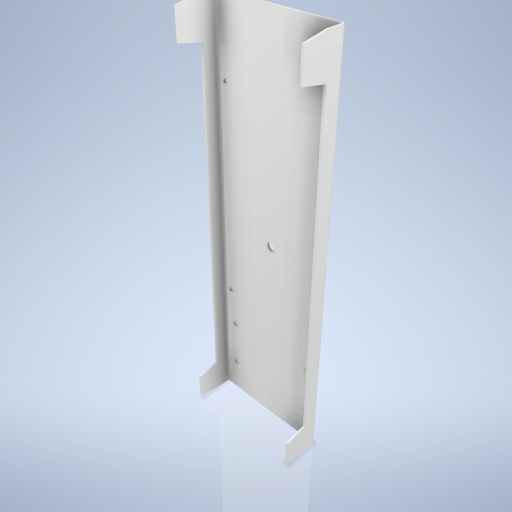
# Autodesk Inventor part: 9
Saved by Autodesk Inventor 2024.2 (Build 282272000, 272)
## iProperties
Created: 2024-05-04
Part Number: 9
Material: Aluminium 6061
Document SubType Name: Sheet Metal
Designer: Fabri
Density: 2.7 g/cm^3
Sheet Metal Rule: Standard_mm
Appearance: Aluminium - flach
Author: Fabri
Autodesk Inventor part; units mm, degrees
note: some values were not read from the file. Chosen so that the rebuilt part matches the saved one: direction of "Bohrung1"; direction of "Bohrung5"; direction of "Bohrung6".
ref_plane "XZ Plane" through (0, 0, 0) normal (0, 1, 0) x (-1, 0, 0)
ref_plane "XY Plane" through (0, 0, 0) normal (0, 0, 1) x (1, 0, 0)
sketch "Skizze1" plane through (0, 0, 0) normal (0, 1, 0) x (-1, 0, 0)
  line L0 (-140, 475) -> (140, 475)
  line L1 (140, 475) -> (140, -475)
  line L2 (140, -475) -> (-140, -475)
  line L3 (-140, -475) -> (-140, 475)
  line L4 (-140, 475) -> (140, -475) construction
  line L5 (140, 475) -> (-140, -475) construction
  point P0 (0, 0)
  dimension "d0" = 950
  dimension "d1" = 280
  measures "d0" distance between parallel lines of L2 L0
  measures "d1" distance between parallel lines of L3 L1
extrude "Grobblech4" add sketch "Skizze1" along normal blind 5
sketch "Skizze2" plane through (140, 0, 475) normal (1, 0, 0) x (0, 1, 0)
  line L0 (0, -950) -> (0, 0)
  line L1 (0, 0) -> (-91, 0)
  line L2 (-91, 0) -> (-91, -950)
  line L3 (-91, -950) -> (0, -950)
  constraints: 6 end point, 1 horizontal, 1 perpendicular, 1 vertical
edge flange "Lasche1" height 96 angle 90 thickness 5 bend radius 5 thickness toward (1, 0, 0) relief tear relief width 5 relief depth 2.5 corner gap 5 corner form 0 edges at (140, 0, 0) (-140, 0, 0) wall of the first edge with corners at (140, 0, -475) (140, 0, 475) (140, -91, 475) (140, -91, -475)
bend "Biegung1"
corner "Ecke1"
sketch "Skizze3" plane through (145, -92.952, 475) normal (1, 0, 0) x (0, 0, -1)
  line L0 (0, 56) -> (10, 1.952)
  line L1 (74, 1.952) -> (84, 56)
  line L2 (84, 56) -> (866, 56)
  line L3 (866, 56) -> (876, 1.952)
  line L4 (876, 1.952) -> (940, 1.952)
  line L5 (940, 1.952) -> (950, 56)
  line L6 (10, 1.952) -> (74, 1.952)
  line L7 (950, 87.952) -> (0, 87.952) projected
  line L8 (0, 1.952) -> (0, 87.952) projected
  line L9 (950, 1.952) -> (0, 1.952) projected
  line L10 (950, 87.952) -> (950, 1.952) projected
  line L11 (950, 1.952) -> (0, 1.952) projected
  point P0 (475, 92.952)
  point P1 (42, 1.952)
  point P2 (908, 1.952)
  point P3 (950, 56)
  point P4 (940, 1.952)
  point P5 (74, 1.952)
  point P6 (876, 1.952)
  point P7 (10, 1.952)
  point P8 (0, 56)
  dimension "d15" = 10
  dimension "d16" = 64
  dimension "d17" = 10
  dimension "d18" = 10
  dimension "d19" = 64
  dimension "d22" = 54.048
  constraints: 14 end point, 3 point on line, 2 midpoint, 1 horizontal alignment, 1 parallel
  measures "d15" horizontal distance of L1.end L1.start
  measures "d16" distance of L1.start L0.end
  measures "d17" horizontal distance of L3.end L2.end
  measures "d18" horizontal distance of L5.end L4.end
  measures "d19" distance of L4.end L3.end
  measures "d22" vertical distance of L4.end L5.end
extrude "Extrusion2" cut sketch "Skizze3" against normal up to surface (5 mm away) contours L0 L9 L8 | L1 L2 L3 L9 | L10 L9 L5
ref_plane "Arbeitsebene1" through (0, 0, 0) normal (1, 0, 0) x (0, 1, 0)
mirror "Spiegeln1" about plane through (0, 0, 0) normal (1, 0, 0) of "Extrusion2"
sketch "Skizze4" plane through (0, 5, 0) normal (0, 1, 0) x (1, 0, 0)
  line L0 (-135, 475) -> (135, 475) projected
  point P0 (110, 391)
  point P1 (-110, 391)
  point P2 (0, 0)
  dimension "d34" = 220
  dimension "d76" = 84
  dimension "d77" = 110
  constraints: 1 horizontal alignment
  measures "d34" distance of point (110, 391) point (-110, 391)
  measures "d76" distance from line of L0 point (110, 391)
  measures "d77" horizontal distance of point (110, 391) point (0, 0)
hole "Bohrung1" at (110, 5, -391) at (-110, 5, -391) direction (0, -1, 0) diameter 12 depth 5
sketch "Skizze5" plane through (0, 5, 0) normal (0, 1, 0) x (1, 0, 0)
  circle A0 centre (-110, 391) radius 6 projected
  point P0 (110, 271)
  point P1 (-110, 271)
  point P2 (110, 391)
  point P3 (0, 0)
  dimension "d43" = 120
  constraints: 2 vertical alignment, 1 horizontal alignment
  measures "d43" distance of point (110, 391) point (110, 271)
hole "Bohrung2" at (110, 5, -271) at (-110, 5, -271) direction (0, -1, 0) diameter 12 end through all
sketch "Skizze6" plane through (0, 5, 0) normal (0, 1, 0) x (1, 0, 0)
  circle A0 centre (110, 271) radius 6 projected
  point P0 (122.5, 176)
  point P1 (-122.5, 176)
  point P2 (0, 0)
  dimension "d55" = 245
  dimension "d88" = 122.5
  dimension "d89" = 95
  constraints: 1 horizontal alignment
  measures "d55" distance of point (122.5, 176) point (-122.5, 176)
  measures "d88" horizontal distance of point (122.5, 176) point (0, 0)
  measures "d89" vertical distance of A0.centre point (122.5, 176)
hole "Bohrung3" at (122.5, 5, -176) at (-122.5, 5, -176) direction (0, -1, 0) diameter 10.106 end through all thread size "M12x1.75" class "6H" standard "ISO Metric profile"
sketch "Skizze7" plane through (0, 5, 0) normal (0, 1, 0) x (1, 0, 0)
  line L0 (145, 475) -> (145, -475) projected
  line L1 (0, 0) -> (0, -582.3396) construction
  point P0 (131, -314)
  point P1 (-124, -314)
  dimension "d73" = 255
  dimension "d79" = 14
  dimension "d80" = 314
  constraints: 2 end point, 1 horizontal alignment, 1 vertical
  measures "d73" distance of point (131, -314) point (-124, -314)
  measures "d79" distance from line of L0 point (131, -314)
  measures "d80" vertical distance of L1.start point (131, -314)
hole "Bohrung5" at (131, 5, 314) at (-124, 5, 314) direction (0, -1, 0) diameter 8.376 depth 5 thread size "M10x1.5" class "6H" standard "ISO Metric profile"
sketch "Skizze8" plane through (0, 5, 0) normal (0, 1, 0) x (1, 0, 0)
  point P0 (0, 0)
  point P1 (0, 0)
  constraints: 1 coincident
hole "Bohrung6" at (0, 5, 0) direction (0, -1, 0) diameter 20 depth 5
equation "\"d31\" = Stärke"
equation "\"d88\" = 0.5 * d55"
equation "\"d64\" = d72"
equation "\"d82\" = d72"
equation "\"d2\" = Stärke"
equation "\"d3\" = BreiteBiegungsfreistellung"
equation "\"d4\" = TiefeBiegungsfreistellung"
equation "\"d5\" = MinimalRest"
equation "\"d6\" = Übergangsradius"
equation "\"d9\" = Biegeradius"
equation "\"d10\" = GrößeEckenfreistellung"
equation "\"d11\" = Abstandsgröße"
equation "\"d12\" = JacobiRadiusGröße"
equation "\"Biegeradius\" = Stärke"
equation "\"BreiteBiegungsfreistellung\" = Stärke"
equation "\"TiefeBiegungsfreistellung\" = 0.5 * Stärke"
equation "\"Übergangsradius\" = Biegeradius"
equation "\"JacobiRadiusGröße\" = Biegeradius"
equation "\"Abstandsgröße\" = Stärke"
equation "\"Stärke\" = 5"
equation "\"d72\" = 107"
equation "\"MinimalRest\" = 10"
equation "\"GrößeEckenfreistellung\" = 20"
